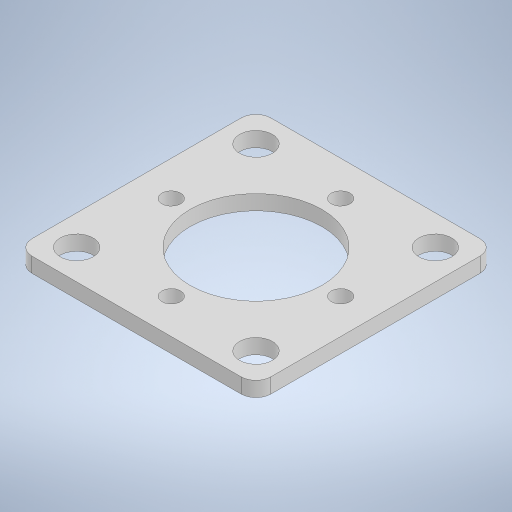
# Autodesk Inventor part: Drive Plate
Saved by Autodesk Inventor 2023.2 (Build 272271000, 271)
## iProperties
Created: 2023-03-16
Part Number: Drive Plate
Material: Generic
Document SubType Name: Modeling
Designer: Nathan Cai
Density: 1 g/cm^3
Appearance: Default
Author: Nathan Cai
Autodesk Inventor part; units mm, degrees
ref_plane "YZ Plane" through (0, 0, 0) normal (1, 0, 0) x (0, 1, 0)
ref_plane "XZ Plane" through (0, 0, 0) normal (0, 1, 0) x (-1, 0, 0)
ref_plane "XY Plane" through (0, 0, 0) normal (0, 0, 1) x (1, 0, 0)
sketch "Sketch1" plane through (0, 0, 0) normal (0, 1, 0) x (-1, 0, 0)
  line L0 (-12.7, 12.7) -> (12.7, 12.7)
  line L1 (12.7, 12.7) -> (12.7, -12.7)
  line L2 (12.7, -12.7) -> (-12.7, -12.7)
  line L3 (-12.7, -12.7) -> (-12.7, 12.7)
  line L4 (-12.7, 12.7) -> (12.7, -12.7) construction
  line L5 (12.7, 12.7) -> (-12.7, -12.7) construction
  line L6 (-9.525, 9.525) -> (9.525, 9.525) construction
  line L7 (9.525, 9.525) -> (9.525, -9.525) construction
  line L8 (9.525, -9.525) -> (-9.525, -9.525) construction
  line L9 (-9.525, -9.525) -> (-9.525, 9.525) construction
  line L10 (-9.525, 9.525) -> (9.525, -9.525) construction
  line L11 (9.525, 9.525) -> (-9.525, -9.525) construction
  circle A0 centre (9.525, 9.525) radius 1.7526
  circle A1 centre (-9.525, 9.525) radius 1.7526
  circle A2 centre (-9.525, -9.525) radius 1.7526
  circle A3 centre (9.525, -9.525) radius 1.7526
  circle A4 centre (0, 0) radius 7
  circle A5 centre (0, 0) radius 9 construction
  line L12 (9, 0) -> (0, 0) construction
  circle A6 centre (9, 0) radius 1
  circle A7 centre (0, 9) radius 1
  circle A8 centre (-9, 0) radius 1
  circle A9 centre (0, -9) radius 1
  dimension "d10" = 18
  dimension "d0" = 25.4
  dimension "d1" = 25.4
  dimension "d2" = 19.05
  dimension "d3" = 19.05
  dimension "d4" = 3.5052
  dimension "d7" = 360
  dimension "d9" = 14
  dimension "d11" = 2
  dimension "d14" = 360
  constraints: 26 end point, 9 centre point, 4 coincident, 4 midpoint, 4 parallel, 3 horizontal, 2 perpendicular, 1 horizontal alignment, 20 other
  measures "d0" distance of L1.end L2.end
  measures "d1" distance of L0.end L1.end
  measures "d2" distance of L7.end L8.end
  measures "d3" distance of L6.end L7.end
  measures "d4" diameter of A0
  measures "d9" diameter of A4
  measures "d11" diameter of A6
extrude "Extrusion1" add sketch "Sketch1" along normal blind 1.5875
fillet "Fillet1" radius 1.5875 4 edges at (-12.7, 0.7937, 12.7) (12.7, 0.7937, 12.7) (-12.7, 0.7937, -12.7) (12.7, 0.7937, -12.7)
body "Solid1"
